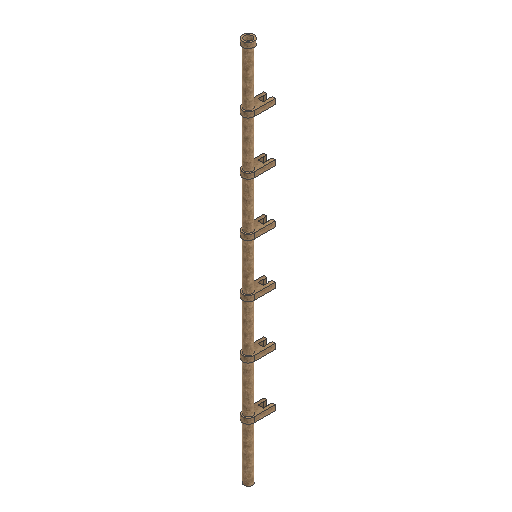
# Autodesk Inventor part: [3DP]bar
Saved by Autodesk Inventor 2024 (Build 280153000, 153)
## iProperties
Created: 2024-04-09
Part Number: [3DP]bar
Material: MDF Medium Density Fiberboard
Document SubType Name: Modeling
Designer: USER
Density: 0.8 g/cm^3
Appearance: Cardboard - Corrugated
Mass: 4.16603 g
Surface Area: 48.6158 cm^2
Volume: 5.20754 cm^3
Author: USER
Autodesk Inventor part; units mm, degrees
ref_plane "YZ Plane" through (0, 0, 0) normal (1, 0, 0) x (0, 1, 0)
ref_plane "XZ Plane" through (0, 0, 0) normal (0, 1, 0) x (-1, 0, 0)
sketch "草圖1" plane through (0, 0, 0) normal (0, 1, 0) x (-1, 0, 0)
  circle A0 centre (0, 0) radius 2.45
  dimension "d0" = 4.9
  constraints: 1 centre point, 1 coincident
  measures "d0" diameter of A0
extrude "擠出1" add sketch "草圖1" along normal blind 215
sketch "草圖2" plane through (0, 215, 0) normal (0, 1, 0) x (1, 0, 0)
  circle A0 centre (0, 0) radius 2.45 projected
  circle A1 centre (0, 0) radius 2.3
  circle A2 centre (0, 0) radius 3.3
  dimension "d3" = 4.6
  dimension "d4" = 6.6
  constraints: 2 centre point, 2 coincident
  measures "d3" diameter of A1
  measures "d4" diameter of A2
extrude "擠出2" add sketch "草圖2" along normal blind 3 contours A0 | A2
ref_plane "工作平面1" through (0, 31, 0) normal (0, -1, 0) x (1, 0, 0)
sketch "草圖3" plane through (0, 31, 0) normal (0, -1, 0) x (1, 0, 0)
  circle A0 centre (0, 0) radius 2.45 projected
  circle A1 centre (0, 0) radius 3.25
  line L0 (3.25, 0) -> (-3.25, 0)
  line L1 (-3.25, 0) -> (-3.25, -12)
  line L2 (-3.25, -12) -> (3.25, -12)
  line L3 (3.25, -12) -> (3.25, 0)
  line L4 (1.6, -12) -> (-1.6, -12)
  line L5 (-1.6, -12) -> (-1.6, -7)
  line L6 (-1.6, -7) -> (1.6, -7)
  line L7 (1.6, -7) -> (1.6, -12)
  line L8 (1.5, -7) -> (-1.5, -7)
  line L9 (-1.5, -7) -> (-1.5, -10)
  line L10 (-1.5, -10) -> (1.5, -10)
  line L11 (1.5, -10) -> (1.5, -7)
  line L12 (1.5, -10) -> (1.2, -10)
  line L13 (1.2, -10) -> (1.6, -12)
  line L14 (-1.5, -10) -> (-1.2, -10)
  line L15 (-1.2, -10) -> (-1.6, -12)
  point P0 (0, -12)
  point P1 (0, -12)
  point P2 (0, -7)
  dimension "d17" = 6.5
  dimension "d9" = 12
  dimension "d11" = 5
  dimension "d12" = 3.2
  dimension "d13" = 3
  dimension "d14" = 3
  dimension "d15" = 0.3
  dimension "d16" = 0.3
  dimension "d18" = 6.5
  constraints: 32 end point, 6 midpoint, 6 parallel, 3 horizontal, 3 perpendicular, 2 coincident, 2 point on line, 1 vertical, 1 vertical alignment, 3 other
  measures "d9" distance of L2.end L0.start
  measures "d11" distance of L6.end L4.start
  measures "d12" distance of L4.start L4.end
  measures "d13" distance of L9.end L10.end
  measures "d14" distance of L10.end L8.start
  measures "d15" distance of L10.end L12.end
  measures "d16" distance of L9.end L14.end
  measures "d18" distance of L1.end L2.end
extrude "擠出3" add sketch "草圖3" against normal blind 3 contours L0 A1 A0 | A0 L0 A1 | L3 L2 L7 L6 L5 L1 A1 | L13 L10 L11 L6 L7 | L5 L6 L9 L10 L15
pattern_linear "矩形陣列1" count 6 spacing 30 along (0, 1, 0) of "擠出3"
